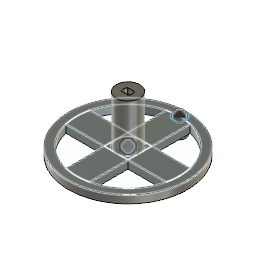
MixingStick_Assembly (Autodesk Fusion 360 archive; units mm, degrees)
design "New Wheel from Hanka Dubovská"
part number: 2026-02-20-08-30-40-446
Autodesk Fusion 360 part; units mm, degrees
sketch "Sketch1" plane through (0, 0, 0) normal (0, 0, 1) x (1, 0, 0)
  circle A0 centre (0, 0) radius 37.5
  circle A1 centre (0, 0) radius 32.5
  circle A2 centre (0, 0) radius 7.5
  line L0 (-2.8, -0.0097) -> (2.8, -0.0097) construction
  arc A3 (-2.0656, 1.8903) -> (-2.0477, -1.9097) centre (0, 0) ccw
  arc A4 (2.0477, -1.9097) -> (2.0656, 1.8903) centre (0, 0) ccw
  line L1 (-2.0656, 1.8903) -> (2.0656, 1.8903)
  line L2 (-2.0477, -1.9097) -> (2.0477, -1.9097)
  arc A5 (-2.0656, 1.8903) -> (-2.0477, -1.9097) centre (0, 0) ccw
  arc A6 (2.0477, -1.9097) -> (2.0656, 1.8903) centre (0, 0) ccw
  line L3 (7.5, -31.6228) -> (7.5, 31.6228)
  line L4 (-7.5, 31.6228) -> (-7.5, -31.6228)
  line L5 (-31.6228, -7.5) -> (31.6228, -7.5)
  line L6 (31.6228, 7.5) -> (-31.6228, 7.5)
  circle A7 centre (-0.0326, 32.5) radius 4
  dimension "d1" = 75
  dimension "d2" = 65
  dimension "d3" = 15
  dimension "d4" = 5.6
  dimension "d43" = 8
  constraint coincident A0.centre A1.centre
  constraint concentric A0 A2
  constraint concentric A2 A3
  constraint coincident L0.start A3
  constraint coincident L0.end A4
  constraint concentric A3 A4
  constraint concentric A0 A5
  constraint horizontal L1
  constraint parallel L1 L2
  constraint concentric A5 A6
  constraint vertical L3
  constraint vertical L4
  constraint coincident A1 L3.end
  constraint coincident A1 L4.end
  constraint tangent A2 L4
  constraint tangent A2 L3
  constraint horizontal L5
  constraint horizontal L6
  constraint coincident A1 L6.start
  constraint coincident A1 L5.start
  constraint tangent A2 L5
  constraint tangent A2 L6
  constraint coincident A1 L6.end
  constraint coincident A1 L5.end
  constraint coincident A1 L3.start
  constraint coincident A1 L4.start
  constraint coincident A1 A7.centre
  measures "d1" diameter of A0
  measures "d2" diameter of A1
  measures "d3" diameter of A2
  measures "d4" diameter of A3
  measures "d43" diameter of A7
extrude "Extrude14" add sketch "Sketch1" against normal blind 12 contours A1 A7 | A1 A7
extrude "Extrude15" add sketch "Sketch1" against normal blind 5 contours A0 | A1 L3 L5 L6 | A1 L3 L4 L6 A7 | A2 L3 L6 | A1 L3 L4 L5 | A2 L3 L5 | A2 | A2 L4 L6 | A2 L4 L5 | A1 L4 L5 L6
extrude "Extrude16" add sketch "Sketch1" along normal blind 30 contours A2
extrude "Extrude17" cut 1 faces at (-1.577, 33.5818, -12) along direction (0, 0, 1) blind 2

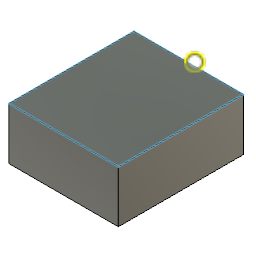
design "body"
part number: 2026-04-21-23-24-45-329
Autodesk Fusion 360 part; units mm, degrees
other "DerivedContext1"
other "DerivedContext2"
sketch "Sketch1" plane through (0.9857, -6.1561, 2.6232) normal (0, 0, 1) x (-1, -0.000039, 0)
  line L0 (1.1997, -145.4227) -> (1.1953, -145.4226)
  line L1 (110.7587, 101.6023) -> (-99.2413, 101.6023)
  line L2 (-99.2413, 101.6023) -> (-99.2413, -138.3977)
  line L3 (-99.2413, -138.3977) -> (110.7587, -138.3977)
  line L4 (110.7587, -138.3977) -> (110.7587, 101.6023)
  dimension "d10" = 210
  dimension "d11" = 240
  constraint horizontal L1
  constraint vertical L2
  constraint horizontal L3
  constraint vertical L4
  measures "d10" distance of L1.start L1.end
  measures "d11" distance of L1.start L3.end
extrude "Extrude4" add sketch "Sketch1" against normal blind 100
shell "Shell1" thickness 5 removed faces 1 at (30.2247, 52.2427, -97.3768)
sketch "sketch 1293" plane through (-0.0052, 132.2416, 0) normal (-0.000039, 1, 0) x (-1, -0.000039, 0)
  line L0 (109.7732, 2.6232) -> (-100.2268, 2.6232)
  line L1 (-100.2268, 2.6232) -> (-100.2268, -97.3768)
  line L2 (-100.2268, -97.3768) -> (109.7732, -97.3768)
  line L3 (109.7732, -97.3768) -> (109.7732, 2.6232)
  line L4 (5, -6) -> (-7.278, -6)
  line L5 (-7.278, -6) -> (-7.278, -0.4131)
  line L6 (-7.278, -0.4131) -> (5, -0.4131)
  line L7 (5, -0.4131) -> (5, -6)
  line L8 (-7.278, -6) -> (-7.278, -0.4131)
  line L9 (-7.278, -0.4131) -> (5, -0.4131)
  line L10 (5, -0.4131) -> (5, -6)
  line L11 (5, -6) -> (-7.278, -6)
extrude "Extrude5" cut sketch "sketch 1293" against normal blind 7 contours L4 L5 L6 L7 L8 L9 L10 L11

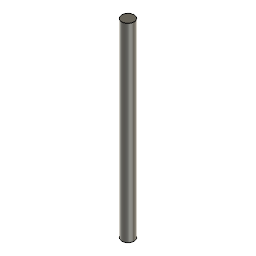
design "motor"
part number: 2026-04-21-23-10-11-437
Autodesk Fusion 360 part; units mm, degrees
other "DerivedContext1"
sketch "Sketch1" plane through (1.0917, -6.231, 19.6232) normal (0, 0, 1) x (-0.999855, -0.017011, 0)
  arc A0 (3.8647, -14.4726) -> (3.976, -10.6742) centre (1.8646, -12.5132) ccw
  line L0 (3.8647, -14.4726) -> (-0.2642, -14.3321)
  arc A1 (-0.1169, -10.5349) -> (-0.2642, -14.3321) centre (1.8646, -12.5132) ccw
  line L1 (-0.1169, -10.5349) -> (3.976, -10.6742)
  circle A2 centre (1.8646, -12.5132) radius 7.5
  circle A3 centre (1.8646, -12.5132) radius 1.2411
  constraint concentric A0 A3
extrude "Extrude1" add sketch "Sketch1" against normal blind 29 contours A3
extrude "Extrude2" add 1 faces at (-0.8278, 5.8662, 19.6232) along direction (0, 0, 1) blind 9

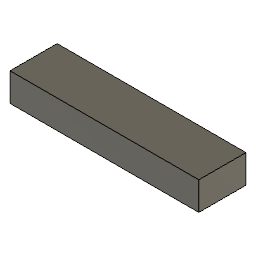
design "Part3"
part number: 2026-05-13-11-13-12-018
Autodesk Fusion 360 part; units mm, degrees
sketch "Sketch1" plane through (0, 0, 0) normal (0, 0, 1) x (1, 0, 0)
  line L0 (25, 230) -> (-15, 230)
  line L1 (-15, 230) -> (-15, 240)
  line L2 (-15, 240) -> (25, 240)
  line L3 (25, 240) -> (25, 230)
  line L4 (10.0636, 232.4278) -> (-0.1364, 232.4278)
  line L5 (-0.1364, 232.4278) -> (-0.1364, 237.6278)
  line L6 (-0.1364, 237.6278) -> (10.0636, 237.6278)
  line L7 (10.0636, 237.6278) -> (10.0636, 232.4278)
  dimension "d1" = 10
  dimension "d2" = 40
  dimension "d3" = 10.2
  dimension "d4" = 5.2
  constraint horizontal L0
  constraint vertical L1
  constraint horizontal L2
  constraint vertical L3
  constraint horizontal L4
  constraint vertical L5
  constraint horizontal L6
  constraint vertical L7
  measures "d1" distance of L0.start L2.end
  measures "d2" distance of L0.start L0.end
  measures "d3" distance of L4.start L4.end
  measures "d4" distance of L4.start L6.end
extrude "Extrude1" add sketch "Sketch1" along normal blind 1 contours L0 L1 L2 L3 | L4 L5 L6 L7
extrude "Extrude2" add sketch "Sketch1" against normal blind 5
extrude "Extrude3" add 1 faces at (11.6667, 233.3333, 1) along direction (0, 0, 1) blind 1
extrude "Extrude4" cut 1 faces at (20.0212, 234.1426, -5) along direction (0, 0, 1) blind 1

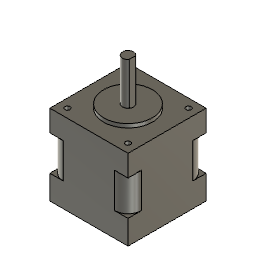
design "StepperMotor"
part number: 2026-04-08-14-01-58-674
Autodesk Fusion 360 part; units mm, degrees
sketch "Sketch1" plane through (0, 0, 0) normal (0, 0, 1) x (1, 0, 0)
  line L0 (0, 0) -> (17.5, 0)
  line L1 (17.5, 0) -> (17.5, 17.5)
  line L2 (17.5, 17.5) -> (0, 17.5)
  line L3 (0, 17.5) -> (0, 0)
  circle A0 centre (3.95, 13.55) radius 1.15
  arc A1 (17.5, 10.9) -> (6.6, 0) centre (17.5, 0) ccw
  arc A2 (17.5, 2.5) -> (15, 0) centre (17.5, 0) ccw
  arc A3 (6, 17.5) -> (0, 11.5) centre (6, 11.5) ccw
  dimension "d1" = 17.5
  dimension "d2" = 17.5
  dimension "d3" = 2.3
  dimension "d4" = 3.95
  dimension "d5" = 3.95
  dimension "d6" = 10.9
  dimension "d7" = 2.5
  dimension "d8" = 6
  dimension "d27" = 6
  constraint coincident L0.start L3.end
  constraint horizontal L0
  constraint perpendicular L0 L1
  constraint perpendicular L1 L2
  constraint perpendicular L0 L3
  constraint coincident L1 A1.start
  constraint coincident L0.end L1.start
  constraint coincident L1 A2.start
  constraint coincident L0 A2.end
  constraint tangent L3 A3
  constraint coincident L2 A3.start
  constraint coincident L3 A3.end
  measures "d1" distance of L0.start L0.end
  measures "d2" distance of L0.end L1.end
  measures "d3" diameter of A0
  measures "d4" distance of L2 A0.centre
  measures "d5" distance of L3 A0.centre
  measures "d6" radius of A1
  measures "d7" radius of A2
  measures "d8" radius of A3
  measures "d27" distance of L2 A3.centre
extrude "Extrude1" add sketch "Sketch1" along normal blind 36 contours L0 L1 L2 L3 A1 A3 | L2 L3 A3
extrude "Extrude2" add sketch "Sketch1" along normal blind 31 contours A0
extrude "Extrude3" add sketch "Sketch1" along normal blind 37.7 contours L0 L1 A1 A2
extrude "Extrude4" add sketch "Sketch1" along normal blind 56.6 contours L0 L1 A2
extrude "Extrude5" cut sketch "Sketch1" along normal blind 15.6 from surface at 10.8 contours L2 L3 A3
mirror "Mirror1" about plane through (15, 0, 0) normal (0, -1, 0) of bodies 1 merged
mirror "Mirror2" about plane through (17.5, 0, 0) normal (1, 0, 0) of bodies 1 merged
sketch "Sketch2" plane through (0, 0, 56.6) normal (0, 0, 1) x (-1, 0, 0)
  circle A0 centre (-17.5, 0) radius 2.5
  circle A1 centre (-17.5, 0) radius 2.5018
  line L0 (-19.5025, -1.4996) -> (-19.5025, 1.4967)
  constraint concentric A0 A1
  constraint coincident A1 L0.start
  constraint coincident A0 L0.end
  constraint vertical L0
extrude "Extrude6" cut sketch "Sketch2" against normal blind 28 contours A0 A1 L0 picked at (-19.5663, -0.4005)

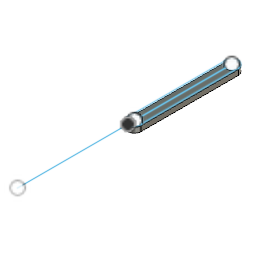
design "Part one"
part number: 2026-04-21-20-15-17-486
Autodesk Fusion 360 part; units mm, degrees
other "DerivedContext1"
sketch "Sketch1" plane through (0, 0, -5) normal (0, 0, -1) x (1, 0, 0)
  circle A0 centre (-0.0164, -32.5205) radius 4.3
  line L0 (4.9902, -32.5205) -> (4.9902, -107.5073)
  line L1 (-5.023, -107.5073) -> (-5.023, -32.5205)
  circle A1 centre (-0.0164, -107.5073) radius 4.3
  arc A2 (-5.023, -107.5073) -> (4.9902, -107.5073) centre (-0.0164, -107.5073) ccw
  arc A3 (4.9902, -32.5205) -> (-5.023, -32.5205) centre (-0.0164, -32.5205) ccw
  line L2 (-0.0164, 57.4861) -> (-0.0164, -112.5139)
  point P0 (-0.0164, -27.5139)
  dimension "d22" = 8.6
  dimension "d25" = 8.6
  dimension "d30" = 170
  constraint vertical L0
  constraint vertical L1
  constraint concentric A0 A3
  constraint tangent L1 A3
  constraint tangent L0 A3
  constraint concentric A1 A2
  constraint tangent L1 A2
  constraint tangent L0 A2
  constraint coincident L0.end A2
  constraint coincident L0 A2.end
  constraint midpoint L2 P0
  constraint coincident A3 P0
  constraint coincident A2 L2.end
  measures "d22" diameter of A0
  measures "d25" diameter of A1
  measures "d30" distance of L2.start L2.end
extrude "Extrude8" add sketch "Sketch1" along normal blind 5 contours A0 L0 A1 A2 A3 L2 | A0 L1 A1 A2 A3 L2
extrude "Extrude9" cut 1 faces at (4.5271, 58.291, -5) along direction (0, 0, -1) blind 1

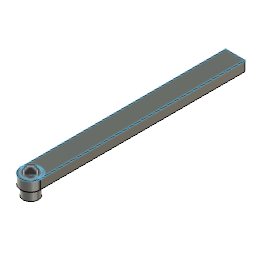
design "Part two"
part number: 2026-04-21-20-33-20-169
Autodesk Fusion 360 part; units mm, degrees
other "DerivedContext1"
sketch "Sketch1" plane through (0, 0, -1) normal (0, 0, 1) x (-1, 0, 0)
  line L0 (5.022, -107.2731) -> (-4.978, -107.2731)
  line L1 (-4.978, -107.2731) -> (-4.978, -212.2731)
  line L2 (-4.978, -212.2731) -> (5.022, -212.2731)
  line L3 (5.022, -212.2731) -> (5.022, -107.2731)
  circle A0 centre (0.0515, -107.4986) radius 4
  circle A1 centre (0.022, -107.2731) radius 5
  dimension "d14" = 10
  dimension "d15" = 105
  dimension "d16" = 8
  constraint horizontal L0
  constraint vertical L1
  constraint horizontal L2
  constraint vertical L3
  constraint midpoint L0 A1.centre
  constraint tangent L3 A1
  measures "d14" distance of L0.start L0.end
  measures "d15" distance of L0.start L2.end
  measures "d16" diameter of A0
extrude "Extrude6" add sketch "Sketch1" against normal blind 5 contours L0 A0 A1 | L0 A0 A1
extrude "Extrude7" add sketch "Sketch1" against normal blind 10 contours L0 A0 | L0 A0
extrude "Extrude8" add sketch "Sketch1" against normal blind 8 contours L1 L2 L3 A1
extrude "Extrude9" add sketch "Sketch1" along normal blind 3 contours L1 L2 L3 A1
extrude "Extrude10" cut 1 faces at (-0.1466, 178.9351, 2) along direction (0, 0, -1) blind 5
extrude "Extrude11" add 1 faces at (-0.1466, 178.9351, -3) along direction (0, 0, 1) blind 2
extrude "Extrude12" cut 1 faces at (-0.1466, 178.9351, -9) along direction (0, 0, 1) blind 3
